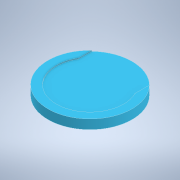
# Autodesk Inventor part: suport senzor
Saved by Autodesk Inventor 2022 (Build 260153000, 153)
## iProperties
Created: 2022-02-27
Part Number: suport senzor
Material: PET Plastic
Document SubType Name: Modeling
Designer: Oana
Density: 1.541 g/cm^3
Appearance: Turquoise
Author: Oana
Autodesk Inventor part; units mm, degrees
ref_plane "YZ Plane" through (0, 0, 0) normal (1, 0, 0) x (0, 1, 0)
ref_plane "XZ Plane" through (0, 0, 0) normal (0, 1, 0) x (-1, 0, 0)
ref_plane "XY Plane" through (0, 0, 0) normal (0, 0, 1) x (1, 0, 0)
sketch "Sketch1" plane through (0, 0, 0) normal (0, 1, 0) x (-1, 0, 0)
  point P0 (0, 0)
sketch "Sketch2" plane through (0, 0, 0) normal (0, 1, 0) x (-1, 0, 0)
  circle A0 centre (0, 0) radius 10
  dimension "d0" = 20
  constraints: 1 centre point, 1 coincident
  measures "d0" diameter of A0
extrude "Extrusion1" add sketch "Sketch2" along normal blind 2
sketch "Sketch3" plane through (0, 2, 0) normal (0, 1, 0) x (1, 0, 0)
  circle A0 centre (0, 0) radius 8
  circle A1 centre (0, 0) radius 10 projected
  dimension "d3" = 2
  constraints: 1 centre point, 1 coincident
  measures "d3" radial gap between concentric circles of A1 A0
extrude "Extrusion2" add sketch "Sketch3" along normal blind 0.2
sketch "Sketch4" plane through (0, 2.2, 0) normal (0, 1, 0) x (1, 0, 0)
  line L0 (-6.842, 3.4953) -> (7.158, 3.4953)
  line L1 (7.158, 3.4953) -> (7.158, 37.4216)
  line L2 (7.158, 37.4216) -> (-6.842, 37.4216)
  line L3 (-6.842, 37.4216) -> (-6.842, 3.4953)
  line L4 (-6.842, 3.4953) -> (7.158, 37.4216) construction
  line L5 (7.158, 3.4953) -> (-6.842, 37.4216) construction
  point P0 (0, 0)
  point P1 (0.158, 20.4584)
  dimension "d6" = 14
  constraints: 12 end point, 2 midpoint, 2 parallel, 1 horizontal, 1 perpendicular
  measures "d6" distance of L2.end L1.end
extrude "Extrusion3" cut sketch "Sketch4" against normal blind 0.2
body "Solid1"
